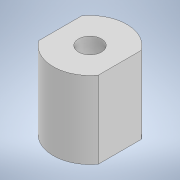
# Autodesk Inventor part: HallSensor_Abstand_8mm4
Saved by Autodesk Inventor 2022.2 (Build 262287010, 287A)
## iProperties
Created: 2024-01-14
Part Number: HallSensor_Abstand_8mm4
Material: Generisch
Document SubType Name: Modeling
Designer: ppovolni
Density: 1 g/cm^3
Appearance: Vorgabe
Author: ppovolni
Autodesk Inventor part; units mm, degrees
ref_plane "YZ Plane" through (0, 0, 0) normal (1, 0, 0) x (0, 1, 0)
ref_plane "XZ Plane" through (0, 0, 0) normal (0, 1, 0) x (-1, 0, 0)
ref_plane "XY Plane" through (0, 0, 0) normal (0, 0, 1) x (1, 0, 0)
sketch "Skizze1" plane through (0, 0, 0) normal (0, 1, 0) x (-1, 0, 0)
  circle A0 centre (0, 0) radius 1.25
  circle A1 centre (0, 0) radius 5 construction
  circle A2 centre (0, 0) radius 4 construction
  line L0 (3.25, -2.3318) -> (3.25, 2.3318)
  line L1 (-3.25, -2.3318) -> (-3.25, 2.3318)
  arc A3 (-3.3811, -2.1373) -> (3.25, -2.3318) centre (0, 0) ccw
  arc A4 (3.3811, 2.1373) -> (-3.3811, 2.1373) centre (0, 0) ccw
  dimension "d2" = 8
  dimension "d0" = 2.5
  dimension "d1" = 10
  dimension "d3" = 6.5
  constraints: 5 coincident, 4 centre point, 4 end point, 4 point on circle, 2 horizontal alignment, 2 vertical, 11 other
  measures "d0" diameter of A0
  measures "d1" diameter of A1
  measures "d3" distance between parallel lines of L0 L1
extrude "Extrusion1" add sketch "Skizze1" along normal blind 8.4
